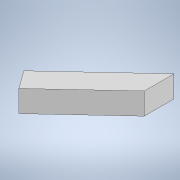
# Autodesk Inventor part: UpperMiniSupport
Saved by Autodesk Inventor 2020.1 (Build 241239000, 239)
## iProperties
Created: 2020-02-04
Part Number: UpperMiniSupport
Material: Generic
Document SubType Name: Modeling
Designer: super
Density: 1 g/cm^3
Appearance: Default
Author: super
Autodesk Inventor part; units mm, degrees
ref_plane "YZ Plane" through (0, 0, 0) normal (1, 0, 0) x (0, 1, 0)
ref_plane "XZ Plane" through (0, 0, 0) normal (0, 1, 0) x (-1, 0, 0)
ref_plane "XY Plane" through (0, 0, 0) normal (0, 0, 1) x (1, 0, 0)
sketch "Sketch1" plane through (0, 0, 0) normal (0, 1, 0) x (-1, 0, 0)
  line L0 (0, 0) -> (22.672, 21.1419)
  line L1 (0, 0) -> (31, 0) construction
  line L2 (22.672, 21.1419) -> (18.9115, 26.3178)
  line L3 (22.672, 21.1419) -> (29.0697, 21.1419) construction
  line L4 (18.9115, 26.3178) -> (0, 8.6825)
  line L5 (0, 8.6825) -> (0, 0)
  dimension "d0" = 31
  dimension "d1" = 43
  dimension "d3" = 126
  constraints: 12 end point, 2 equal length, 2 horizontal, 1 parallel, 1 perpendicular
  measures "d0" distance of L0.start L0.end
  measures "d1" angle of L1 L0
  measures "d3" angle of L3 L2
extrude "Extrusion1" add sketch "Sketch1" along normal blind 6.35
body "Solid1"
